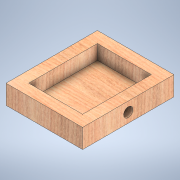
# Autodesk Inventor part: MADERA
Saved by Autodesk Inventor 2022.6 (Build 266554000, 554)
## iProperties
Created: 2025-01-14
Part Number: MADERA
Material: Genérico
Document SubType Name: Modeling
Designer: johan
Density: 1 g/cm^3
Appearance: Valor por defecto
Author: johan
Autodesk Inventor part; units mm, degrees
ref_plane "YZ Plane" through (0, 0, 0) normal (1, 0, 0) x (0, 1, 0)
ref_plane "XZ Plane" through (0, 0, 0) normal (0, 1, 0) x (-1, 0, 0)
ref_plane "XY Plane" through (0, 0, 0) normal (0, 0, 1) x (1, 0, 0)
sketch "Boceto2" plane through (0, 0, 0) normal (0, 1, 0) x (-1, 0, 0)
  line L0 (0, 0) -> (243, 0)
  line L1 (243, 0) -> (243, -290)
  line L2 (243, -290) -> (0, -290)
  line L3 (0, -290) -> (0, 0)
  dimension "d4" = 243
  dimension "d5" = 290
  constraints: 8 end point, 2 parallel, 1 horizontal, 1 perpendicular
  measures "d4" distance of L1.end L2.end
  measures "d5" distance of L0.end L1.end
extrude "Extrusión2" add sketch "Boceto2" along normal blind 61
sketch "Boceto3" plane through (0, 61, 0) normal (0, 1, 0) x (1, 0, 0)
  line L0 (0, 290) -> (-243, 290) projected
  line L1 (-243, 290) -> (-243, 0) projected
  line L2 (-243, 0) -> (0, 0) projected
  line L3 (0, 0) -> (0, 290) projected
  line L4 (-207, 36) -> (-207, 254)
  line L5 (-207, 254) -> (-36, 254)
  line L6 (-36, 254) -> (-36, 36)
  line L7 (-36, 36) -> (-207, 36)
  dimension "d8" = 36
  constraints: 8 end point, 3 other
  measures "d8" distance between parallel lines of L1 L4
sketch "Boceto4" plane through (0, 0, 0) normal (1, 0, 0) x (0, 0, -1)
  line L0 (0, 0) -> (290, 0) projected
  line L1 (290, 0) -> (290, 61) projected
  line L2 (0, 61) -> (290, 61) projected
  line L3 (0, 0) -> (0, 61) projected
  circle A0 centre (145, 30.5) radius 14.78
  dimension "d9" = 29.56
  constraints: 1 centre point
  measures "d9" diameter of A0
extrude "Extrusión3" cut sketch "Boceto4" against normal blind 69.75 contours A0
extrude "Extrusión4" cut sketch "Boceto3" against normal blind 46.25 contours L4 L5 L6 L7
